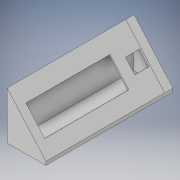
# Autodesk Inventor part: Suport - pantalla i potenciometre
Saved by Autodesk Inventor 2019 (Build 230136000, 136)
## iProperties
Created: 2018-08-18
Part Number: Suport - pantalla i potenciometre
Material: Genérico
Document SubType Name: Modeling
Designer: Albert Garangou Culebras
Density: 1 g/cm^3
Appearance: Valor por defecto
Author: Albert Garangou Culebras
Autodesk Inventor part; units mm, degrees
ref_plane "YZ Plane" through (0, 0, 0) normal (1, 0, 0) x (0, 1, 0)
ref_plane "XZ Plane" through (0, 0, 0) normal (0, 1, 0) x (-1, 0, 0)
ref_plane "XY Plane" through (0, 0, 0) normal (0, 0, 1) x (1, 0, 0)
sketch "Boceto3" plane through (0, 0, 0) normal (0, 0, 1) x (1, 0, 0)
  line L0 (40, 0) -> (37, 0)
  line L1 (0, 0) -> (0, 45)
  line L2 (0, 45) -> (3, 45)
  line L3 (40, 0) -> (40, 3)
  line L4 (40, 3) -> (3, 45)
  line L5 (0, 0) -> (40, 0)
  dimension "d3" = 3
  dimension "d4" = 45
  dimension "d5" = 3
  dimension "d6" = 3
  constraints: 12 end point, 2 horizontal, 2 vertical, 1 perpendicular
  measures "d3" distance of L0.start L0.end
  measures "d4" distance of L1.start L1.end
  measures "d5" distance of L1.end L2.end
  measures "d6" distance of L0.start L3.end
extrude "Extrusión1" add sketch "Boceto3" against normal blind 98.2
sketch "Boceto4" plane through (0, 0, 0) normal (0, 0, 1) x (1, 0, 0)
  line L0 (3.3154, 41.6201) -> (2, 43)
  line L1 (3.3154, 41.6201) -> (38, 2)
  line L2 (38, 2) -> (2, 2)
  line L3 (2, 2) -> (2, 43)
  point P0 (0, 45)
  constraints: 8 end point, 1 horizontal
extrude "Extrusión2" cut sketch "Boceto4" against normal blind 210.55
sketch "Boceto6" plane through (0, 0, 0) normal (0, 0, 1) x (1, 0, 0)
  line L0 (1.0395, 0.9992) -> (39.0395, 0.9992)
  line L1 (39.0395, 1.0003) -> (39.0395, 1.9993) projected
  line L2 (39.0395, 0.9992) -> (39.0395, 1.9993)
  line L3 (39.0395, 1.9993) -> (3, 44.0003)
  line L4 (2.88, 44.0003) -> (1, 44.0003) projected
  line L5 (3, 44.0003) -> (1, 44.0003)
  line L6 (1, 1.0003) -> (39.0395, 1.0003) projected
  line L7 (1, 44.0003) -> (1, 1.0003)
  point P0 (0, 0)
  constraints: 10 end point, 2 perpendicular, 1 horizontal, 1 parallel
extrude "Extrusión3" add sketch "Boceto6" against normal blind 2
sketch "Boceto7" plane through (0, 0, -98.2) normal (0, 0, -1) x (-1, 0, 0)
  line L0 (-1, 1.0003) -> (-39.0395, 1.0003) projected
  line L1 (-1, 1.0003) -> (-39.0395, 1.0003)
  line L2 (-39.0395, 1.0003) -> (-39.0395, 2)
  line L3 (-39.0395, 1.9993) -> (-2.88, 44.0003) projected
  line L4 (-39.0395, 2) -> (-2.88, 44.0003)
  line L5 (-2.88, 44.0003) -> (-1, 44.0003) projected
  line L6 (-1, 44.0003) -> (-1, 1.0003)
  line L7 (-2.88, 44.0003) -> (6.9067, 55.3678)
  line L8 (6.9067, 55.3678) -> (10.1689, 59.157)
  line L9 (10.1689, 59.157) -> (10.1689, 0)
  line L10 (10.1689, 0) -> (0, 0)
  dimension "d68" = 15
  dimension "d70" = 5
  constraints: 17 end point, 2 perpendicular, 2 vertical, 1 collinear
  measures "d68" distance of L3.end L7.end
  measures "d70" distance of L7.end L8.end
extrude "Extrusión4" add sketch "Boceto7" against normal blind 2
sketch "Boceto10" plane through (0, 0, -96.2) normal (0, 0, 1) x (1, 0, 0)
  line L0 (20.1691, 1.0003) -> (21.6691, 1.0003)
  line L1 (39.0395, 1.0003) -> (1, 1.0003) projected
  line L2 (21.6691, 1.0003) -> (21.6691, 22.1759)
  line L3 (2.88, 44.0003) -> (39.0395, 1.9993) projected
  line L4 (21.6691, 22.1759) -> (20.1691, 23.9182)
  line L5 (20.1691, 23.9182) -> (20.1691, 1.0003)
  point P0 (0, 0)
  dimension "d49" = 1.5
  constraints: 8 end point, 2 point on line, 1 collinear, 1 parallel, 1 vertical
  measures "d49" distance of L0.start L0.end
extrude "Extrusión7" add sketch "Boceto10" along normal blind 96
sketch "Boceto15" plane through (0, 0, -98.2) normal (0, 0, -1) x (-1, 0, 0)
  line L0 (-3, 45) -> (-40, 3) projected
  line L1 (-20.3927, 25.257) -> (-7.1721, 40.2641)
  line L2 (-7.1721, 40.2641) -> (-7.1721, 0)
  line L3 (-20.1691, 1.0003) -> (-1, 1.0003) projected
  line L4 (-7.1721, 40.2641) -> (-3, 45)
  line L5 (0, 45) -> (-3, 45)
  line L6 (0, 0) -> (0, 45) projected
  line L7 (0, 45) -> (0, 0)
  line L8 (0, 0) -> (-7.1721, 0)
  line L9 (-40, 0) -> (0, 0) projected
  dimension "d71" = 20
  constraints: 12 end point, 3 collinear, 2 point on line, 1 horizontal, 1 perpendicular
  measures "d71" distance of L1.start L1.end
extrude "Extrusión9" cut sketch "Boceto15" against normal blind 617.4
sketch "Boceto16" plane through (0, 0, -96.2) normal (0, 0, 1) x (1, 0, 0)
  line L0 (7.1721, 1) -> (8.6721, 1.0003)
  line L1 (20.1691, 1.0003) -> (7.1721, 1.0003) projected
  line L2 (8.6721, 1.0003) -> (8.6721, 37.2725)
  line L3 (7.1721, 39.0149) -> (20.1691, 23.9182) projected
  line L4 (8.6721, 37.2725) -> (7.1721, 39.0149)
  line L5 (7.1721, 39.0149) -> (7.1721, 1)
  point P0 (0, 0)
  dimension "d74" = 1.5
  constraints: 8 end point, 1 collinear, 1 parallel, 1 perpendicular, 1 point on line
  measures "d74" distance of L0.start L0.end
extrude "Extrusión10" add sketch "Boceto16" along normal blind 95.4
sketch "Boceto17" plane through (0, 0, 0) normal (0, 0, 1) x (1, 0, 0)
  line L0 (20.1691, 1.0003) -> (8.6721, 1.0003) projected
  line L1 (8.6721, 35.5011) -> (8.6721, 2) projected
  line L2 (8.6721, 1.0003) -> (8.6721, 37.2725)
  line L3 (39.0395, 1.9993) -> (21.6691, 22.1759) projected
  line L4 (8.6721, 37.2725) -> (39.0395, 1.9993)
  line L5 (39.0395, 1.9993) -> (39.0395, 1.0003)
  line L6 (39.0395, 1.0003) -> (8.6721, 1.0003)
  line L7 (40, 0) -> (7.1721, 0) projected
  point P0 (0, 0)
  constraints: 8 end point, 2 collinear, 2 parallel
extrude "Extrusión11" cut sketch "Boceto17" against normal blind 235.6
sketch "Boceto21" plane through (40, 3, 0) normal (0.750359, 0.6610305, 0) x (0, 0, -1)
  line L0 (5, 24.1901) -> (5, 36.1901)
  line L1 (5, 36.1901) -> (5, 12.1901)
  line L2 (5, 12.1901) -> (76, 12.1901)
  line L3 (76, 12.1901) -> (76, 36.1901)
  line L4 (76, 36.1901) -> (5, 36.1901)
  line L5 (85, 24.1901) -> (85, 18.1901)
  line L6 (85, 18.1901) -> (91, 18.1901)
  line L7 (91, 18.1901) -> (97, 18.1901)
  line L8 (97, 18.1901) -> (97, 30.1901)
  line L9 (97, 30.1901) -> (85, 30.1901)
  line L10 (85, 30.1901) -> (85, 24.1901)
  line L11 (76, 24.1901) -> (81, 24.1901)
  line L12 (81, 24.1901) -> (85, 24.1901)
  point P0 (0, 24.1901)
  dimension "d114" = 5
  constraints: 26 end point, 6 perpendicular, 3 point on line, 2 horizontal, 1 midpoint
  measures "d114" distance of L11.end L11.start
extrude "Extrusión13" cut sketch "Boceto21" against normal blind 1.5
sketch "Boceto22" plane through (0, 0, 0) normal (0, 0, 1) x (1, 0, 0)
  line L0 (8.6721, 1.0003) -> (39.0395, 1.0003) projected
  line L1 (8.6721, 1.0003) -> (39.0395, 1.0003)
  line L2 (39.0395, 1.0003) -> (39.0395, 2)
  line L3 (39.0395, 2) -> (8.6721, 37)
  line L4 (8.6721, 37.2725) -> (8.6721, 1.0003) projected
  line L5 (8.6721, 37) -> (8.6721, 1.0003)
  line L6 (7.1721, 0) -> (7.1721, 40.2641) projected
  line L7 (7.1721, 40.2641) -> (7.1721, 0)
  line L8 (40, 3) -> (40, 0) projected
  line L9 (7.1721, 0) -> (40, 0)
  line L10 (40, 0) -> (40, 3)
  line L11 (40, 3) -> (7.1721, 40.2641)
  line L12 (7.1721, 40.2641) -> (40, 3) projected
  point P0 (0, 0)
  constraints: 16 end point, 3 collinear, 3 perpendicular, 1 horizontal
extrude "Extrusión14" add sketch "Boceto22" along normal blind 2
sketch "Boceto24" plane through (0, 0, 2) normal (0, 0, 1) x (1, 0, 0)
  line L0 (8.6721, 1.0003) -> (8.6721, 37) projected
  line L1 (39.0395, 1.0003) -> (8.6721, 1.0003) projected
  line L2 (8.6721, 1.0003) -> (39.0395, 1.0003)
  line L3 (39.0395, 1.0003) -> (39.0395, 2)
  line L4 (39.0395, 2) -> (8.6721, 37)
  line L5 (8.6721, 37) -> (8.6721, 1.0003)
  point P0 (0, 0)
  constraints: 8 end point, 1 collinear, 1 parallel, 1 perpendicular
extrude "Extrusión15" add sketch "Boceto24" against normal blind 2
sketch "Boceto25" plane through (0, 0, -98.2) normal (0, 0, -1) x (-1, 0, 0)
  line L0 (-8.6721, 1.0003) -> (-8.6721, 37.2725) projected
  line L1 (-8.6721, 1.0003) -> (-8.6721, 37.2725)
  line L2 (-8.6721, 37.2725) -> (-39, 2)
  line L3 (-39, 2) -> (-39, 1.0003)
  line L4 (-39, 1.0003) -> (-8.6721, 1.0003)
  line L5 (-7.1721, 0) -> (-40, 0) projected
  line L6 (-7.1721, 40) -> (-7.1721, 0)
  line L7 (-40, 0) -> (-7.1721, 0)
  line L8 (-40, 0) -> (-40, 2.8598)
  line L9 (-7.1721, 0) -> (-7.1721, 40.2641) projected
  line L10 (-40, 2.8598) -> (-7.1721, 40.2641)
  point P0 (0, 0)
  constraints: 16 end point, 2 parallel, 2 vertical, 1 collinear, 1 perpendicular
extrude "Extrusión16" add sketch "Boceto25" along normal blind 7
sketch "Boceto27" plane through (0, 0, -105.2) normal (0, 0, -1) x (-1, 0, 0)
  line L0 (-8.6721, 1.0003) -> (-39.0395, 1.0003) projected
  line L1 (-8.6721, 1.0003) -> (-39.0395, 1.0003)
  line L2 (-39.0395, 1.0003) -> (-39.0395, 1.9993)
  line L3 (-8.6721, 1.0003) -> (-8.6721, 37.2725) projected
  line L4 (-39.0395, 1.9993) -> (-8.6721, 37.2725)
  line L5 (-8.6721, 37.2725) -> (-8.6721, 1.0003)
  point P0 (0, 0)
  constraints: 8 end point, 2 collinear, 1 perpendicular
extrude "Extrusión17" add sketch "Boceto27" against normal blind 2
